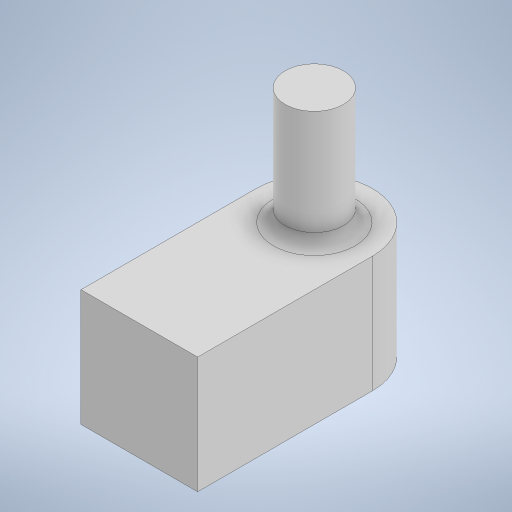
# Autodesk Inventor part: 05-17-2023 cardine inferiore analisi fem
Saved by Autodesk Inventor 2023 (Build 270158000, 158)
## iProperties
Created: 2023-05-17
Part Number: 05-17-2023 cardine inferiore analisi fem
Material: Generico
Document SubType Name: Modeling
Designer: Admin
Density: 1 g/cm^3
Appearance: Default
Author: Admin
Autodesk Inventor part; units mm, degrees
ref_plane "YZ Plane" through (0, 0, 0) normal (1, 0, 0) x (0, 1, 0)
ref_plane "XZ Plane" through (0, 0, 0) normal (0, 1, 0) x (-1, 0, 0)
ref_plane "XY Plane" through (0, 0, 0) normal (0, 0, 1) x (1, 0, 0)
sketch "Schizzo1" plane through (0, 0, 0) normal (0, 1, 0) x (-1, 0, 0)
  line L0 (10, 20) -> (-10, 20)
  line L1 (-10, 20) -> (-10, -20)
  line L2 (-10, -20) -> (10, -20)
  line L3 (10, -20) -> (10, 20)
  line L4 (10, 20) -> (-10, -20) construction
  line L5 (-10, 20) -> (10, -20) construction
  point P0 (0, 0)
  dimension "d0" = 40
  dimension "d1" = 20
  constraints: 12 end point, 2 midpoint, 2 parallel, 1 horizontal, 1 perpendicular
  measures "d0" distance of L2.end L0.start
  measures "d1" distance between parallel lines of L1 L3
extrude "Estrusione1" add sketch "Schizzo1" along normal blind 20
sketch "Schizzo2" plane through (0, 20, 0) normal (0, 1, 0) x (1, 0, 0)
  line L0 (0, 0) -> (0, 10)
  circle A0 centre (0, 10) radius 5
  dimension "d4" = 10
  dimension "d5" = 10
  constraints: 2 end point, 1 centre point, 1 coincident, 1 vertical
  measures "d4" distance of L0.start L0.end
  measures "d5" diameter of A0
extrude "Estrusione2" add sketch "Schizzo2" along normal blind 20
fillet "Raccordo1" radius 10 2 edges at (10, 10, -20) (-10, 10, -20)
fillet "Raccordo2" radius 2 1 edges at (-5, 20, -10)
